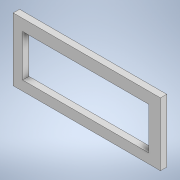
# Autodesk Inventor part: mouth_open
Saved by Autodesk Inventor 2021 (Build 250183000, 183)
## iProperties
Created: 2023-06-07
Part Number: mouth_open
Material: Generic
Document SubType Name: Modeling
Designer: LENOVO
Density: 1 g/cm^3
Appearance: Default
Author: LENOVO
Autodesk Inventor part; units mm, degrees
ref_plane "YZ Plane" through (0, 0, 0) normal (1, 0, 0) x (0, 1, 0)
ref_plane "XZ Plane" through (0, 0, 0) normal (0, 1, 0) x (-1, 0, 0)
ref_plane "XY Plane" through (0, 0, 0) normal (0, 0, 1) x (1, 0, 0)
sketch "Sketch1" plane through (0, 0, 0) normal (0, 0, 1) x (1, 0, 0)
  line L0 (-7.1091, 0) -> (62.8909, 0)
  line L1 (62.8909, 0) -> (62.8909, -30)
  line L2 (62.8909, -30) -> (-7.1091, -30)
  line L3 (-7.1091, -30) -> (-7.1091, 0)
  point P0 (0, 0)
  dimension "d0" = 70
  dimension "d1" = 30
  constraints: 8 end point, 2 parallel, 1 horizontal, 1 perpendicular
  measures "d0" distance of L1.end L2.end
  measures "d1" distance of L0.end L1.end
extrude "Extrusion1" add sketch "Sketch1" along normal blind 3
sketch "Sketch2" plane through (0, 0, 3) normal (0, 0, 1) x (1, 0, 0)
  line L0 (57.3616, -25.4008) -> (-2.6384, -25.4008)
  line L1 (-2.6384, -25.4008) -> (-2.6384, -5.4008)
  line L2 (-2.6384, -5.4008) -> (57.3616, -5.4008)
  line L3 (57.3616, -5.4008) -> (57.3616, -25.4008)
  line L4 (57.3616, -25.4008) -> (-2.6384, -5.4008) construction
  line L5 (-2.6384, -25.4008) -> (57.3616, -5.4008) construction
  point P0 (0, 0)
  point P1 (27.3616, -15.4008)
  dimension "d4" = 60
  dimension "d5" = 20
  constraints: 12 end point, 2 midpoint, 2 parallel, 1 horizontal, 1 perpendicular
  measures "d4" distance of L1.end L2.end
  measures "d5" distance of L0.end L1.end
extrude "Extrusion2" cut sketch "Sketch2" against normal blind 3
body "Solid1"
